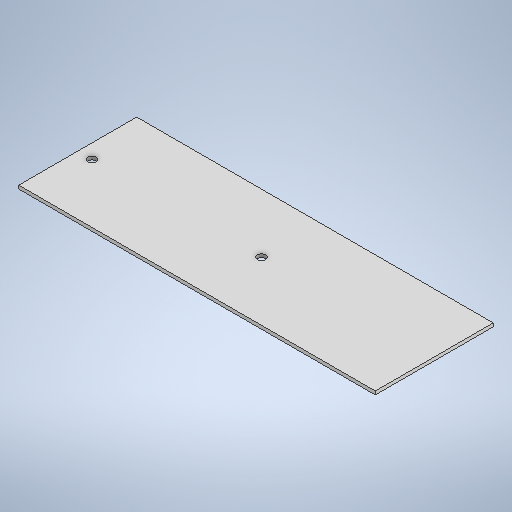
# Autodesk Inventor part: Board
Saved by Autodesk Inventor 2025 (Build 290162010, 162A)
## iProperties
Created: 2024-06-06
Part Number: Board
Material: Generic
Document SubType Name: Modeling
Designer: vncnt
Density: 1 g/cm^3
Appearance: Default
Author: vncnt
Autodesk Inventor part; units mm, degrees
ref_plane "YZ Plane" through (0, 0, 0) normal (1, 0, 0) x (0, 1, 0)
ref_plane "XZ Plane" through (0, 0, 0) normal (0, 1, 0) x (-1, 0, 0)
ref_plane "XY Plane" through (0, 0, 0) normal (0, 0, 1) x (1, 0, 0)
sketch "Sketch1" plane through (0, 0, 0) normal (0, 1, 0) x (-1, 0, 0)
  line L0 (0, 0) -> (-165.1, 0)
  line L1 (-165.1, 0) -> (-165.1, -54.61)
  line L2 (-165.1, -54.61) -> (0, -54.61)
  line L3 (0, -54.61) -> (0, 0)
  circle A0 centre (-6.604, -27.305) radius 1.905
  circle A1 centre (-85.09, -27.305) radius 1.905
  dimension "d0" = 165.1
  dimension "d1" = 54.61
  dimension "d2" = 27.305
  dimension "d3" = 6.604
  dimension "d4" = 3.81
  dimension "d5" = 78.486
  dimension "d8" = 3.81
  constraints: 8 end point, 2 centre point, 2 parallel, 1 horizontal, 1 perpendicular
  measures "d0" distance of L1.end L2.end
  measures "d1" distance of L2.end L0.start
  measures "d2" distance from line of L2 A0.centre
  measures "d3" distance from line of L3 A0.centre
  measures "d4" diameter of A0
  measures "d5" distance of A1.centre A0.centre
  measures "d8" diameter of A1
extrude "Extrusion1" add sketch "Sketch1" along normal blind 1.58
body "Solid1"
